gear-encoder v14 (Autodesk Fusion 360 design; units mm, degrees)
description: Spur Gear; Module: 0.4; Num Teeth: 11; Pressure Angle: 20.0; Backlash: 0.00 mm
Autodesk Fusion 360 part; units mm, degrees
sketch "スケッチ1" plane through (0, 0, 0) normal (0, 0, 1) x (1, 0, 0) in component "Spur Gear (11 teeth)"
  circle A0 centre (0, 0) radius 1.6692
  circle A1 centre (0, 0) radius 0.75
extrude "押し出し1" add sketch "スケッチ1" along normal blind 1 in component "Spur Gear (11 teeth)"
sketch "スケッチ2" plane through (0, 0, 0) normal (0, 0, 1) x (1, 0, 0) in component "Spur Gear (11 teeth)"
  spline S0 degree 3 poles (2.0417, -0.3247) (2.0617, -0.3252) (2.1023, -0.3263) (2.1635, -0.3166) (2.2253, -0.3024) (2.2875, -0.283) (2.3498, -0.259) (2.4123, -0.2307) (2.4745, -0.1982) (2.5366, -0.1618) (2.5768, -0.1347) (2.5972, -0.1211) knots 0 0 0 0 0.005994 0.012164 0.018504 0.025015 0.031695 0.038544 0.045564 0.052752 0.060111 0.060111 0.060111 0.060111
  spline S1 degree 3 poles (2.0417, 0.3247) (2.0617, 0.3252) (2.1023, 0.3263) (2.1635, 0.3166) (2.2253, 0.3024) (2.2875, 0.283) (2.3498, 0.259) (2.4123, 0.2307) (2.4745, 0.1982) (2.5366, 0.1618) (2.5768, 0.1347) (2.5972, 0.1211) knots 0 0 0 0 0.005994 0.012164 0.018504 0.025015 0.031695 0.038544 0.045564 0.052752 0.060111 0.060111 0.060111 0.060111
  arc A0 (2.5972, -0.1211) -> (2.5972, 0.1211) centre (0, 0) ccw
  line L0 (1.6386, -0.2621) -> (2.0417, -0.3247)
  line L1 (1.6386, 0.2621) -> (2.0417, 0.3247)
  line L2 (1.6386, -0.2621) -> (1.6386, 0.2621)
  point P0 (2.1016, -0.3245)
  point P1 (2.1627, -0.316)
  point P2 (2.2245, -0.3018)
  point P3 (2.2867, -0.2825)
  point P4 (2.3491, -0.2586)
  point P5 (2.4115, -0.2303)
  point P6 (2.4737, -0.1979)
  point P7 (2.5357, -0.1615)
  point P8 (2.1016, 0.3245)
  point P9 (2.1627, 0.316)
  point P10 (2.2245, 0.3018)
  point P11 (2.2867, 0.2825)
  point P12 (2.3491, 0.2586)
  point P13 (2.4115, 0.2303)
  point P14 (2.4737, 0.1979)
  point P15 (2.5357, 0.1615)
extrude "押し出し2" add sketch "スケッチ2" along normal blind 1 in component "Spur Gear (11 teeth)"
pattern_circular "C パターン1" count 11 over 360 about axis through (0, 0, 0) along (0, 0, 1) of "押し出し2" in component "Spur Gear (11 teeth)"
sketch "スケッチ3" plane through (0, 0, 0) normal (0, 0, 1) x (1, 0, 0) in component "Spur Gear (11 teeth)"
  circle A0 centre (0, 0) radius 2.2 construction
component "Spur Gear (11 teeth)" placed x (1, 0, 0) y (0, 1, 0) z (0, 0, 1) at (0, 0, 0)
